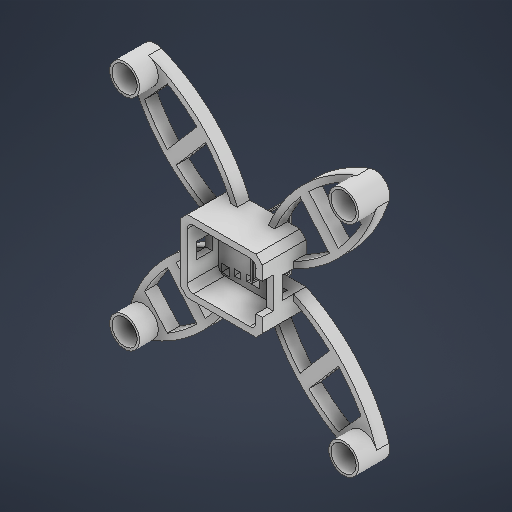
# Autodesk Inventor part: Frame1
Saved by Autodesk Inventor 2027 (Build 310192000, 192)
## iProperties
Created: 2026-07-11
Part Number: Frame1
Material: Genérico
Document SubType Name: Modeling
Designer: marcu
Mass: 8.18846 g
Surface Area: 101.647 cm^2
Volume: 8.18846 cm^3
Density: 1 g/cm^3
Appearance: Padrão
Author: marcu
Autodesk Inventor part; units mm, degrees
ref_plane "YZ Plane" through (0, 0, 0) normal (1, 0, 0) x (0, 1, 0)
ref_plane "XZ Plane" through (0, 0, 0) normal (0, 1, 0) x (-1, 0, 0)
sketch "Esboço1" plane through (0, 0, 0) normal (0, 0, 1) x (1, 0, 0)
  line L0 (-11, 9.5) -> (11, 9.5)
  line L1 (11, 9.5) -> (11, -9.5)
  line L2 (11, -9.5) -> (-11, -9.5)
  line L3 (-11, -9.5) -> (-11, 9.5)
  line L4 (-11, 9.5) -> (11, -9.5) construction
  line L5 (11, 9.5) -> (-11, -9.5) construction
  line L6 (-13, 11.5) -> (13, 11.5)
  line L7 (13, 11.5) -> (13, -11.5)
  line L8 (13, -11.5) -> (-13, -11.5)
  line L9 (-13, -11.5) -> (-13, 11.5)
  line L10 (-13, 11.5) -> (13, -11.5) construction
  line L11 (13, 11.5) -> (-13, -11.5) construction
  line L12 (-35, 35) -> (35, 35) construction
  line L13 (35, 35) -> (35, -35) construction
  line L14 (35, -35) -> (-35, -35) construction
  line L15 (-35, -35) -> (-35, 35) construction
  line L16 (-35, 35) -> (35, -35) construction
  line L17 (35, 35) -> (-35, -35) construction
  circle A0 centre (35, 35) radius 4
  circle A1 centre (35, 35) radius 4.75
  circle A2 centre (35, 35) radius 3
  line L18 (0, 0) -> (0, 20) construction
  line L19 (0, 0) -> (-19.2045, 0) construction
  circle A3 centre (-35, 35) radius 4
  circle A4 centre (-35, 35) radius 4.75
  circle A5 centre (-35, 35) radius 3
  line L20 (-35, -35) -> (35, -35) construction
  circle A6 centre (35, -35) radius 4
  circle A7 centre (35, -35) radius 4.75
  circle A8 centre (35, -35) radius 3
  circle A9 centre (-35, -35) radius 3
  circle A10 centre (-35, -35) radius 4
  circle A11 centre (-35, -35) radius 4.75
  line L21 (-7, 11.5) -> (-7, 18.6053) construction
  line L22 (5, 11.5) -> (5, 18.6053) construction
  arc A12 (33.2807, 39.4279) -> (5, 11.5) centre (51.3788, -7.1817) ccw
  line L23 (13, 3.5) -> (19, 3.5) construction
  arc A13 (13, 3.5) -> (39.5224, 33.5474) centre (-8.0821, 48.8381) ccw
  line L24 (7, 11.5) -> (7, 16) construction
  line L25 (13, 5.5) -> (16.0625, 5.5) construction
  arc A14 (30.4046, 36.2021) -> (7, 11.5) centre (52.8319, -8.4859) ccw
  arc A15 (13, 5.5) -> (36.4791, 30.4861) centre (-9.4889, 50.157) ccw
  line L26 (-13, 3.5) -> (-19, 3.5) construction
  line L27 (-7, 11.5) -> (-7, 16) construction
  line L28 (-13, 5.5) -> (-16.0625, 5.5) construction
  line L29 (-7, -11.5) -> (-7, -18.6053) construction
  line L30 (5, -11.5) -> (5, -18.6053) construction
  line L31 (13, -3.5) -> (19, -3.5) construction
  line L32 (7, -11.5) -> (7, -16) construction
  line L33 (13, -5.5) -> (16.0625, -5.5) construction
  line L34 (-7, -11.5) -> (-7, -16) construction
  line L35 (-13, -5.5) -> (-16.0625, -5.5) construction
  line L36 (-13, -3.5) -> (-19, -3.5) construction
  arc A16 (-39.5224, 33.5474) -> (-13, 3.5) centre (8.0821, 48.8381) ccw
  arc A17 (-36.4791, 30.4861) -> (-13, 5.5) centre (9.4889, 50.157) ccw
  arc A18 (39.5224, -33.5474) -> (13, -3.5) centre (-8.0821, -48.8381) ccw
  arc A19 (36.4791, -30.4861) -> (13, -5.5) centre (-9.4889, -50.157) ccw
  arc A20 (5, -11.5) -> (33.2807, -39.4279) centre (51.3788, 7.1817) ccw
  arc A21 (7, -11.5) -> (30.4046, -36.2021) centre (52.8319, 8.4859) ccw
  arc A22 (-13, -3.5) -> (-39.5224, -33.5474) centre (8.0821, -48.8381) ccw
  arc A23 (-13, -5.5) -> (-36.4791, -30.4861) centre (9.4889, -50.157) ccw
  line L37 (-5, 11.5) -> (-5, 15.8149) construction
  line L38 (-5, -11.5) -> (-5, -15.6696) construction
  arc A24 (-5, 11.5) -> (-33.2807, 39.4279) centre (-51.3788, -7.1817) ccw
  arc A25 (-7, 11.5) -> (-30.4046, 36.2021) centre (-52.8319, -8.4859) ccw
  arc A26 (-33.2807, -39.4279) -> (-5, -11.5) centre (-51.3788, 7.1817) ccw
  arc A27 (-30.4046, -36.2021) -> (-7, -11.5) centre (-52.8319, 8.4859) ccw
  line L39 (24.4858, 13.473) -> (15.1366, 24.3632)
  line L40 (27.3177, 16.3151) -> (17.8987, 27.2866)
  line L41 (24.4858, -13.473) -> (15.1366, -24.3632)
  line L42 (27.3177, -16.3151) -> (17.8987, -27.2866)
  line L43 (-24.4858, 13.473) -> (-15.1366, 24.3632)
  line L44 (-27.3177, 16.3151) -> (-17.8987, 27.2866)
  line L45 (-24.4858, -13.473) -> (-15.1366, -24.3632)
  line L46 (-27.3177, -16.3151) -> (-17.8987, -27.2866)
  line L47 (34.5822, 26.5407) -> (27.3271, 34.52)
  line L48 (34.5822, -26.5407) -> (27.3271, -34.52)
  line L49 (-34.5822, 26.5407) -> (-27.3271, 34.52)
  line L50 (-34.5822, -26.5407) -> (-27.3271, -34.52)
  point P0 (-13, 5.5)
  point P1 (-13, 3.5)
  point P2 (-13, -5.5)
  point P3 (-13, -3.5)
  point P4 (13, -5.5)
  point P5 (13, -3.5)
  point P6 (7, -11.5)
  point P7 (5, -11.5)
  point P8 (-7, 11.5)
  point P9 (-7, -11.5)
  point P10 (-24.4858, 13.473)
  point P11 (-15.1366, 24.3632)
  point P12 (-17.8987, 27.2866)
  point P13 (-27.3177, 16.3151)
  point P14 (17.8987, -27.2866)
  point P15 (27.3177, -16.3151)
  point P16 (24.4858, -13.473)
  point P17 (15.1366, -24.3632)
  point P18 (-27.3177, -16.3151)
  point P19 (-17.8987, -27.2866)
  point P20 (-15.1366, -24.3632)
  point P21 (-24.4858, -13.473)
  point P22 (27.3271, -34.52)
  point P23 (-34.5822, 26.5407)
  point P24 (-27.3271, 34.52)
  point P25 (-27.3271, -34.52)
  point P26 (-34.5822, -26.5407)
  dimension "d0" = 22
  dimension "d1" = 19
  dimension "d2" = 26
  dimension "d3" = 23
  dimension "d4" = 70
  dimension "d5" = 70
  dimension "d6" = 8
  dimension "d7" = 9.5
  dimension "d8" = 6
  dimension "d9" = 8
  dimension "d10" = 6
  dimension "d11" = 50
  dimension "d12" = 6
  dimension "d13" = 8
  dimension "d14" = 50
  dimension "d15" = 6
  dimension "d16" = 6
  dimension "d17" = 50
  dimension "d18" = 50
  dimension "d21" = 50
  dimension "d22" = 50
  dimension "d23" = 50
  dimension "d24" = 50
  dimension "d25" = 50
  dimension "d26" = 50
  dimension "d29" = 50
  dimension "d30" = 50
  dimension "d44" = 8
  dimension "d45" = 8
  dimension "d46" = 50
  dimension "d47" = 50
  dimension "d48" = 50
  dimension "d49" = 50
  dimension "d76" = 18
  dimension "d77" = 22
  dimension "d78" = 10
  dimension "d79" = 14
  dimension "d120" = 6
  dimension "d121" = 26.0867
  constraints: 102 end point, 54 point on circle, 49 symmetric about line, 28 centre point, 16 tangent, 12 coincident, 7 point on line, 6 midpoint, 6 parallel, 5 horizontal, 5 perpendicular, 5 vertical, 9 other
  measures "d0" distance of L1.end L2.end
  measures "d1" distance of L0.end L1.end
  measures "d2" distance of L7.end L8.end
  measures "d3" distance of L6.end L7.end
  measures "d4" distance between parallel lines of L14 L12
  measures "d5" distance between parallel lines of L15 L13
  measures "d6" diameter of A0
  measures "d7" diameter of A1
  measures "d8" diameter of A2
  measures "d9" distance from line of L6.end L22
  measures "d10" distance from line of L6.start L21
  measures "d11" radius of A12
  measures "d12" distance of L23.start L23.end
  measures "d13" distance from line of L6.end L23
  measures "d14" radius of A13
  measures "d15" distance from line of L6.end L24
  measures "d16" distance from line of L6.end L25
  measures "d17" radius of A14
  measures "d18" radius of A15
  measures "d21" radius of A16
  measures "d22" radius of A17
  measures "d23" radius of A18
  measures "d24" radius of A19
  measures "d25" radius of A20
  measures "d26" radius of A21
  measures "d29" radius of A22
  measures "d30" radius of A23
  measures "d44" distance from line of L6.start L37
  measures "d45" distance from line of L8.end L38
  measures "d46" radius of A24
  measures "d47" radius of A25
  measures "d48" radius of A26
  measures "d49" radius of A27
  measures "d76" distance from line of A1.centre L40
  measures "d77" distance from line of A1.centre L39
  measures "d78" distance from line of L6.end L39
  measures "d79" distance from line of L40 L6.end
  measures "d120" distance from line of A1.centre L47
  measures "d121" distance from line of L47 L6.end
extrude "Extrusão1" add sketch "Esboço1" along normal blind 14 contours L6 L7 L8 L9
extrude "Extrusão2" add sketch "Esboço1" along normal blind 4 contours L0 L1 L2 L3
extrude "Extrusão3" add sketch "Esboço1" along normal blind 4 contours A25 A4 A24 L6 | L9 A16 A4 A17 | L43 A17 L44 A25 | A12 A1 A14 L6 | L9 A23 A11 A22 | A25 L49 A17 A4 | A14 L40 A15 L39 | A1 A15 L47 A14 | L45 A27 L46 A23 | A23 L50 A27 A11 | A11 A27 L8 A26 | A15 A1 A13 L7 | L8 A21 A7 A20 | A18 A7 A19 L7 | L41 A19 L42 A21 | A21 L48 A19 A7
extrude "Extrusão4" add sketch "Esboço1" along normal blind 10 contours A4 | A1 | A11 | A7
extrude "Extrusão5" add sketch "Esboço1" along normal blind 2 contours A0 | A3 | A6 | A10
sketch "Esboço2" plane through (13, -11.5, 14) normal (1, 0, 0) x (0, 0, -1)
  line L0 (14, 15) -> (14, 8) projected
  line L1 (14, 8) -> (6.5, 8)
  line L2 (6.5, 8) -> (6.5, 15)
  line L3 (6.5, 15) -> (14, 15)
  line L4 (14, 15) -> (14, 8)
  point P0 (14, 11.5)
  point P1 (14, 15)
  dimension "d132" = 7
  dimension "d133" = 7.5
  constraints: 8 end point, 2 parallel, 1 horizontal, 1 perpendicular
  measures "d132" distance of L2.end L1.end
  measures "d133" distance of L3.end L2.end
sketch "Esboço3" plane through (0, 0, 14) normal (0, 0, 1) x (1, 0, 0)
  line L0 (11, -5) -> (13, -5)
  line L1 (13, -5) -> (13, 5)
  line L2 (13, 5) -> (11, 5)
  line L3 (11, 5) -> (11, -5)
  line L4 (11, -5) -> (13, 5) construction
  line L5 (13, -5) -> (11, 5) construction
  line L6 (-11, -9.5) -> (-11, 9.5) projected
  line L7 (13, 11.5) -> (-13, 11.5) projected
  point P0 (0, 0)
  point P1 (12, 0)
  dimension "d54" = 10
  dimension "d57" = 24
  dimension "d58" = 22
  dimension "d59" = 6.5
  constraints: 12 end point, 2 midpoint, 2 parallel, 1 horizontal, 1 perpendicular
  measures "d54" distance of L1.end L0.end
  measures "d57" distance between parallel lines of L6 L1
  measures "d58" distance between parallel lines of L6 L3
  measures "d59" distance between parallel lines of L7 L2
extrude "Extrusão7" cut sketch "Esboço3" against normal blind 3.5
chamfer "Chanfro2" distance 2 angle 45 4 edges at (13, 11.5, 7) (-13, 11.5, 7) (13, -11.5, 7) (-13, -11.5, 7)
fillet "Arredondamento1" radius 2 4 edges at (-11, -9.5, 9) (-11, 9.5, 9) (11, -9.5, 9) (11, 9.5, 9)
sketch "Esboço4" plane through (0, 0, 4) normal (0, 0, 1) x (1, 0, 0)
  line L0 (-6, -8) -> (-4, -8)
  line L1 (-4, -8) -> (-4, -6)
  line L2 (-4, -6) -> (-6, -6)
  line L3 (-6, -6) -> (-6, -8)
  line L4 (-6, -8) -> (-4, -6) construction
  line L5 (-4, -8) -> (-6, -6) construction
  line L6 (9, -9.5) -> (-9, -9.5) projected
  line L7 (-11, -7.5) -> (-11, 7.5) projected
  line L8 (0, 0) -> (-2.75, 0) construction
  line L9 (-2, -7.5) -> (2, -7.5)
  line L10 (2, -7.5) -> (2, -5.5)
  line L11 (2, -5.5) -> (-2, -5.5)
  line L12 (-2, -5.5) -> (-2, -7.5)
  line L13 (-2, -7.5) -> (2, -5.5) construction
  line L14 (2, -7.5) -> (-2, -5.5) construction
  line L15 (-6, 8) -> (-4, 8)
  line L16 (-4, 8) -> (-4, 6)
  line L17 (-4, 6) -> (-6, 6)
  line L18 (-6, 6) -> (-6, 8)
  line L19 (-6, 8) -> (-4, 6) construction
  line L20 (-4, 8) -> (-6, 6) construction
  line L21 (-2, 7.5) -> (2, 7.5)
  line L22 (2, 7.5) -> (2, 5.5)
  line L23 (2, 5.5) -> (-2, 5.5)
  line L24 (-2, 5.5) -> (-2, 7.5)
  line L25 (-2, 7.5) -> (2, 5.5) construction
  line L26 (2, 7.5) -> (-2, 5.5) construction
  point P0 (-5, -7)
  point P1 (0, -6.5)
  point P2 (-5, 7)
  point P3 (0, 6.5)
  dimension "d66" = 2
  dimension "d67" = 2
  dimension "d68" = 1.5
  dimension "d69" = 5
  dimension "d70" = 4
  dimension "d71" = 2
  dimension "d72" = 2
  dimension "d73" = 2
  constraints: 50 end point, 10 symmetric about line, 4 midpoint, 4 parallel, 3 horizontal, 2 perpendicular
  measures "d66" distance of L2.end L1.end
  measures "d67" distance of L1.end L0.end
  measures "d68" distance between parallel lines of L0 L6
  measures "d69" distance between parallel lines of L3 L7
  measures "d70" distance of L11.end L10.end
  measures "d71" distance of L10.end L9.end
  measures "d72" distance between parallel lines of L6 L9
  measures "d73" distance between parallel lines of L12 L1
extrude "Extrusão8" cut sketch "Esboço4" against normal blind 5
sketch "Esboço7" plane through (-13, -3.5, 0) normal (-1, 0, 0) x (0, 0, 1)
  line L0 (11, 6) -> (6, 6)
  line L1 (6, 6) -> (6, 1)
  line L2 (6, 1) -> (11, 1)
  line L3 (11, 1) -> (11, 6)
  line L4 (11, 6) -> (6, 1) construction
  line L5 (6, 6) -> (11, 1) construction
  line L6 (14, 13) -> (14, -6) projected
  line L7 (0, 13) -> (14, 13) projected
  point P0 (0, 3.5)
  point P1 (8.5, 3.5)
  dimension "d114" = 5
  dimension "d115" = 5
  dimension "d116" = 3
  dimension "d117" = 7
  constraints: 12 end point, 2 midpoint, 2 parallel, 1 horizontal, 1 perpendicular
  measures "d114" distance of L2.end L1.end
  measures "d115" distance of L1.end L0.end
  measures "d116" distance between parallel lines of L6 L3
  measures "d117" distance between parallel lines of L7 L0
extrude "Extrusão11" cut sketch "Esboço7" against normal blind 5
sketch "Esboço8" plane through (0, 0, 0) normal (0, 0, -1) x (-1, 0, 0)
  circle A0 centre (17.2758, 24.9417) radius 1.15
  line L0 (24.4858, 13.473) -> (15.1366, 24.3632) projected
  arc A1 (33.2807, 39.4279) -> (5, 11.5) centre (51.3788, -7.1817) ccw projected
  circle A2 centre (25.1293, 15.7938) radius 1.15
  arc A3 (13, 3.5) -> (39.5224, 33.5474) centre (-8.0821, 48.8381) ccw projected
  line L1 (0, 0) -> (16.246, 0) construction
  line L2 (16.246, 0) -> (0, 0) construction
  line L3 (0, 0) -> (0, 18.9105) construction
  circle A4 centre (17.2758, -24.9417) radius 1.15
  line L4 (24.4858, -13.473) -> (15.1366, -24.3632)
  circle A5 centre (25.1293, -15.7938) radius 1.15
  circle A6 centre (-17.2758, 24.9417) radius 1.15
  circle A7 centre (-25.1293, 15.7938) radius 1.15
  circle A8 centre (-17.2758, -24.9417) radius 1.15
  circle A9 centre (-25.1293, -15.7938) radius 1.15
  dimension "d122" = 2.3
  dimension "d123" = 2
  dimension "d125" = 2.3
  dimension "d126" = 2
  dimension "d128" = 2
  dimension "d129" = 2
  constraints: 8 centre point, 8 end point, 8 symmetric about line, 1 collinear, 1 horizontal, 1 vertical, 6 other
  measures "d122" diameter of A0
  measures "d123" distance from line of A0.centre L0
  measures "d125" diameter of A2
  measures "d126" distance from line of L0 A2.centre
extrude "Extrusão12" cut sketch "Esboço8" against normal blind 2
extrude "Extrusão13" cut sketch "Esboço2" against normal blind 12
ref_plane "Plano de trabalho1" through (0, 0, 4.5) normal (0, 0, 1) x (1, 0, 0)
sketch "Esboço9" plane through (0, 0, 4.5) normal (0, 0, 1) x (1, 0, 0)
  line L0 (0.25, -6.75) -> (-0.25, -6.75)
  line L1 (-0.25, -6.75) -> (-0.25, -6.25)
  line L2 (-0.25, -6.25) -> (0.25, -6.25)
  line L3 (0.25, -6.25) -> (0.25, -6.75)
  line L4 (-2, -7.5) -> (-2, -5.5) projected
  line L5 (0, 0) -> (-1.8899, 0) construction
  line L6 (0.25, 6.75) -> (-0.25, 6.75)
  line L7 (-0.25, 6.75) -> (-0.25, 6.25)
  line L8 (-0.25, 6.25) -> (0.25, 6.25)
  line L9 (0.25, 6.25) -> (0.25, 6.75)
  dimension "d138" = 0.5
  dimension "d139" = 0.5
  dimension "d140" = 6.25
  dimension "d141" = 1.75
  constraints: 18 end point, 4 symmetric about line, 2 horizontal, 2 parallel, 1 perpendicular
  measures "d138" distance of L0.start L0.end
  measures "d139" distance of L0.end L1.end
  measures "d140" distance from line of L5.start L2
  measures "d141" distance between parallel lines of L4 L1
sketch3d "Esboço 3D3"
  line L0 (0.25, -6.75, 4.5) -> (0.25, -6.75, 0)
  line L1 (0.25, -6.75, 0) -> (0.25, -10.5, 0)
  line L2 (0.25, -10.5, 0) -> (0.25, -10.5, -8)
  line L3 (0.25, -10.5, -8) -> (0.25, 10.5, -8)
  line L4 (0.25, 10.5, -8) -> (0.25, 10.5, 0)
  line L5 (0.25, 10.5, 0) -> (0.25, 6.75, 0)
  line L6 (0.25, 6.75, 0) -> (0.25, 6.75, 4.5)
  line L7 (0.25, 6.75, 4.5) -> (0.25, -6.75, 4.5)
  dimension "d150" = 4.5
  dimension "d151" = 3.75
  dimension "d152" = 8
  dimension "d153" = 4.5
  dimension "d154" = 3.75
  dimension "d155" = 8
sweep "Enforca_gato" add profiles "Esboço9" path "Esboço 3D3" contours L0 L1 L2 L3
sketch "Esboço10" plane through (0, 0, 4) normal (0, 0, 1) x (1, 0, 0)
  line L0 (7.5, -9) -> (10, -9)
  line L1 (10, -9) -> (10, -6.5)
  line L2 (10, -6.5) -> (7.5, -6.5)
  line L3 (7.5, -6.5) -> (7.5, -9)
  line L4 (9, -9.5) -> (-9, -9.5) projected
  line L5 (0, 0) -> (-4, 0) construction
  line L6 (7.5, 9) -> (10, 9)
  line L7 (10, 9) -> (10, 6.5)
  line L8 (10, 6.5) -> (7.5, 6.5)
  line L9 (7.5, 6.5) -> (7.5, 9)
  line L10 (0, 0) -> (0, 8.2642) construction
  line L11 (0.25, -10) -> (0.25, 10) projected
  line L12 (-7.5, -9) -> (-10, -9)
  line L13 (-10, -9) -> (-10, -6.5)
  line L14 (-10, -6.5) -> (-7.5, -6.5)
  line L15 (-7.5, -6.5) -> (-7.5, -9)
  line L16 (-7.5, 6.5) -> (-7.5, 9)
  line L17 (-7.5, 9) -> (-10, 9)
  line L18 (-10, 9) -> (-10, 6.5)
  line L19 (-10, 6.5) -> (-7.5, 6.5)
  dimension "d160" = 2.5
  dimension "d161" = 2.5
  dimension "d162" = 7.5
  dimension "d163" = 0.5
  constraints: 36 end point, 12 symmetric about line, 3 parallel, 2 horizontal, 1 perpendicular
  measures "d160" distance of L2.end L1.end
  measures "d161" distance of L1.end L0.end
  measures "d162" distance from line of L5.start L3
  measures "d163" distance between parallel lines of L4 L0
extrude "Extrusão14" cut sketch "Esboço10" against normal blind 10
sketch "Esboço11" plane through (0, 0, 4) normal (0, 0, 1) x (1, 0, 0)
  point P0 (0, 0)
